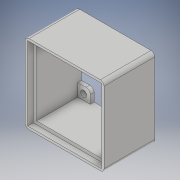
# Autodesk Inventor part: camerashield
Saved by Autodesk Inventor 2019 (Build 230136000, 136)
## iProperties
Created: 2019-07-22
Part Number: camerashield
Material: Generic
Document SubType Name: Modeling
Designer: Dell
Density: 1 g/cm^3
Appearance: Default
Author: Dell
Autodesk Inventor part; units mm, degrees
ref_plane "YZ Plane" through (0, 0, 0) normal (1, 0, 0) x (0, 1, 0)
ref_plane "XZ Plane" through (0, 0, 0) normal (0, 1, 0) x (-1, 0, 0)
ref_plane "XY Plane" through (0, 0, 0) normal (0, 0, 1) x (1, 0, 0)
sketch "Sketch1" plane through (0, 0, 0) normal (0, 0, 1) x (1, 0, 0)
  line L0 (-21, -21) -> (21, -21)
  line L1 (21, -21) -> (21, 21)
  line L2 (21, 21) -> (-21, 21)
  line L3 (-21, 21) -> (-21, -21)
  line L4 (-21, -21) -> (21, 21) construction
  line L5 (21, -21) -> (-21, 21) construction
  line L6 (-18, -18) -> (18, -18)
  line L7 (18, -18) -> (18, 18)
  line L8 (18, 18) -> (-18, 18)
  line L9 (-18, 18) -> (-18, -18)
  line L10 (-18, -18) -> (18, 18) construction
  line L11 (18, -18) -> (-18, 18) construction
  line L12 (18, 18) -> (13.26, 18)
  line L13 (13.26, 18) -> (13.26, 13.26)
  line L14 (13.26, 13.26) -> (18, 13.26)
  line L15 (18, 13.26) -> (18, 18)
  line L16 (18, 18) -> (14.885, 18)
  line L17 (14.885, 18) -> (14.885, 14.885)
  line L18 (14.885, 14.885) -> (18, 14.885)
  line L19 (18, 14.885) -> (18, 18)
  circle A0 centre (14.885, 14.885) radius 1.625
  line L20 (18, 18) -> (11.3, 18)
  line L21 (11.3, 18) -> (11.3, 11.3)
  line L22 (11.3, 11.3) -> (18, 11.3)
  line L23 (18, 11.3) -> (18, 18)
  circle A1 centre (13.26, 13.26) radius 1.96
  point P0 (0, 0)
  dimension "d0" = 42
  dimension "d1" = 42
  dimension "d2" = 36
  dimension "d3" = 36
  dimension "d4" = 4.74
  dimension "d5" = 4.74
  dimension "d6" = 3.115
  dimension "d7" = 6.7
  dimension "d8" = 6.7
  constraints: 48 end point, 10 parallel, 5 horizontal, 5 perpendicular, 4 midpoint, 2 centre point, 2 coincident, 1 point on line, 1 tangent
  measures "d0" distance of L2.end L1.end
  measures "d1" distance of L0.end L1.end
  measures "d2" distance of L8.end L7.end
  measures "d3" distance of L6.end L7.end
  measures "d4" distance of L14.end L13.end
  measures "d5" distance of L12.end L13.end
  measures "d6" distance of L18.end L17.end
  measures "d7" distance of L22.end L21.end
  measures "d8" distance of L20.end L21.end
extrude "Extrusion1" add sketch "Sketch1" along normal blind 2 contours L3 L2 L1 L0 | L22 A1 L14 L7 | L8 L13 A1 L21 | L14 A1 A0 L18 L7 | L22 L21 A1 | A1 L13 L14 | L8 L17 A0 A1 L13 | L18 A0 L17 L8 L7 | L14 A0 A1 | A1 A0 L13 | A0 A1 L17 L18 | L18 L17 A0 | L14 L13 A0 | A0 A1
mirror "Mirror1" about plane through (0, 0, 0) normal (1, 0, 0) of "Extrusion1"
mirror "Mirror2" about plane through (0, 0, 0) normal (0, 1, 0) of "Extrusion1", "Mirror1"
fillet "Fillet1" radius 2.25 4 edges at (-11.3, 11.3, 1) (11.3, 11.3, 1) (11.3, -11.3, 1) (-11.3, -11.3, 1)
sketch "Sketch2" plane through (0, 0, 2) normal (0, 0, 1) x (1, 0, 0)
  line L0 (21, -21) -> (21, 21) projected
  line L1 (21, 21) -> (14.885, 21)
  line L2 (14.885, 21) -> (14.885, 14.885)
  line L3 (14.885, 14.885) -> (21, 14.885)
  line L4 (21, 14.885) -> (21, 21)
  circle A0 centre (14.885, 14.885) radius 1.625
  point P0 (0, 0)
  dimension "d12" = 6.115
  dimension "d13" = 6.115
  dimension "d14" = 3.25
  constraints: 8 end point, 2 parallel, 1 centre point, 1 coincident, 1 horizontal, 1 perpendicular
  measures "d12" distance of L3.end L2.end
  measures "d13" distance of L1.end L2.end
  measures "d14" diameter of A0
extrude "Extrusion2" cut sketch "Sketch2" against normal blind 2 contours A0 L2 L3 | L3 L2 A0
mirror "Mirror3" about plane through (0, 0, 0) normal (0, 1, 0) of "Extrusion2"
mirror "Mirror4" about plane through (0, 0, 0) normal (1, 0, 0) of "Extrusion2", "Mirror3"
sketch "Sketch3" plane through (0, 0, 2) normal (0, 0, 1) x (1, 0, 0)
  line L0 (-18, -18) -> (18, -18)
  line L1 (18, -18) -> (18, 18)
  line L2 (18, 18) -> (-18, 18)
  line L3 (-18, 18) -> (-18, -18)
  line L4 (-18, -18) -> (18, 18) construction
  line L5 (18, -18) -> (-18, 18) construction
  line L6 (21, 21) -> (-21, 21) projected
  line L7 (-21, -21) -> (21, -21)
  line L8 (21, -21) -> (21, 21)
  line L9 (21, 21) -> (-21, 21)
  line L10 (-21, 21) -> (-21, -21)
  line L11 (-21, -21) -> (21, 21) construction
  line L12 (21, -21) -> (-21, 21) construction
  point P0 (0, 0)
  dimension "d17" = 36
  dimension "d18" = 36
  constraints: 24 end point, 4 midpoint, 4 parallel, 2 horizontal, 2 perpendicular
  measures "d17" distance of L2.end L1.end
  measures "d18" distance of L0.end L1.end
extrude "Extrusion3" add sketch "Sketch3" along normal blind 22
sketch "Sketch4" plane through (0, 0, 24) normal (0, 0, 1) x (1, 0, 0)
  line L0 (21, 21) -> (-21, 21) projected
  line L1 (-21, -21) -> (21, -21)
  line L2 (21, -21) -> (21, 21)
  line L3 (21, 21) -> (-21, 21)
  line L4 (-21, 21) -> (-21, -21)
  line L5 (-21, -21) -> (21, 21) construction
  line L6 (21, -21) -> (-21, 21) construction
  line L7 (-19.7, -19.7) -> (19.7, -19.7)
  line L8 (19.7, -19.7) -> (19.7, 19.7)
  line L9 (19.7, 19.7) -> (-19.7, 19.7)
  line L10 (-19.7, 19.7) -> (-19.7, -19.7)
  line L11 (-19.7, -19.7) -> (19.7, 19.7) construction
  line L12 (19.7, -19.7) -> (-19.7, 19.7) construction
  point P0 (0, 0)
  dimension "d21" = 39.4
  dimension "d22" = 39.4
  constraints: 24 end point, 4 midpoint, 4 parallel, 2 horizontal, 2 perpendicular
  measures "d21" distance of L9.end L8.end
  measures "d22" distance of L7.end L8.end
extrude "Extrusion4" add sketch "Sketch4" along normal blind 3
fillet "Fillet2" radius 2 4 edges at (21, -21, 13.5) (21, 21, 13.5) (-21, 21, 13.5) (-21, -21, 13.5)
body "Solid1"
